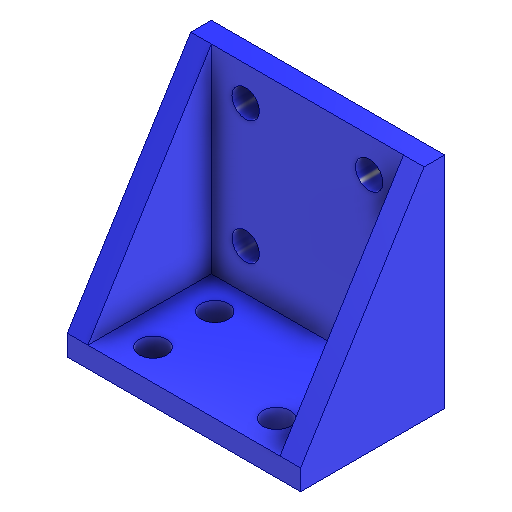
# Autodesk Inventor part: Escuadra
Saved by Autodesk Inventor 2025.3 (Build 293356000, 356)
## iProperties
Created: 2025-10-28
Part Number: Escuadra
Material: ABS Plastic
Document SubType Name: Modeling
Designer: Gabriel Bojaca
Density: 1.06 g/cm^3
Appearance: Blue - Wall Paint - Glossy
Author: Gabriel Bojaca
Title: Escuadra.ipt
Autodesk Inventor part; units mm, degrees
ref_plane "YZ Plane" through (0, 0, 0) normal (1, 0, 0) x (0, 1, 0)
ref_plane "XZ Plane" through (0, 0, 0) normal (0, 1, 0) x (-1, 0, 0)
ref_plane "XY Plane" through (0, 0, 0) normal (0, 0, 1) x (1, 0, 0)
sketch "Sketch1" plane through (0, 0, 0) normal (0, 0, 1) x (1, 0, 0)
  line L0 (-9, -9) -> (9, -9) construction
  line L1 (9, -9) -> (9, 9) construction
  line L2 (9, 9) -> (-9, 9) construction
  line L3 (-9, 9) -> (-9, -9) construction
  line L4 (-9, -9) -> (9, 9) construction
  line L5 (9, -9) -> (-9, 9) construction
  circle A0 centre (-9, 9) radius 2
  circle A1 centre (9, 9) radius 2
  circle A2 centre (9, -9) radius 2
  circle A3 centre (-9, -9) radius 2
  line L6 (-13.4025, 9) -> (21.0308, 9) construction
  line L7 (-13.4025, -18) -> (21.0308, -18)
  line L8 (14, -14) -> (-14, -14)
  line L9 (-14, -14) -> (-14, 14)
  line L10 (-14, 14) -> (14, 14)
  line L11 (14, 14) -> (14, -14)
  line L12 (-14, 14) -> (14, 14)
  line L13 (14, 14) -> (14, -18)
  line L14 (14, -18) -> (-14, -18)
  line L15 (-14, -18) -> (-14, 14)
  point P0 (0, 0)
  dimension "d0" = 18
  dimension "d1" = 18
  dimension "d2" = 4
  dimension "d3" = 4
  dimension "d4" = 27
  dimension "d5" = 5
  dimension "d6" = 9
  dimension "d7" = 14
  constraints: 32 end point, 7 parallel, 4 centre point, 3 horizontal, 3 perpendicular, 2 coincident, 2 midpoint, 2 symmetric about line, 1 point on line, 5 other
  measures "d0" distance of L2.end L1.end
  measures "d1" distance of L1.end L0.end
  measures "d2" diameter of A0
  measures "d3" diameter of A1
  measures "d4" distance between parallel lines of L6 L7
  measures "d5" distance between parallel lines of L0 L8
  measures "d6" distance from line of point (0, 0) L6
  measures "d7" distance from line of L9 point (0, 0)
extrude "Extrusion1" add sketch "Sketch1" along normal blind 3
sketch "Sketch2" plane through (-14, -18, 0) normal (0, -1, 0) x (1, 0, 0)
  line L0 (0, 3) -> (28, 3)
  line L1 (28, 3) -> (28, 21)
  line L2 (28, 21) -> (0, 21)
  line L3 (0, 21) -> (0, 3)
  line L4 (0, 21) -> (28, 3) construction
  line L5 (5, 7.5) -> (23, 7.5) construction
  line L6 (23, 7.5) -> (23, 16.5) construction
  line L7 (23, 16.5) -> (5, 16.5) construction
  line L8 (5, 16.5) -> (5, 7.5) construction
  line L9 (5, 7.5) -> (23, 16.5) construction
  line L10 (23, 7.5) -> (5, 16.5) construction
  circle A0 centre (5, 16.5) radius 2
  circle A1 centre (23, 16.5) radius 2
  line L11 (5, 12) -> (23, 12) construction
  line L12 (14, 16.5) -> (14, 7.5) construction
  circle A2 centre (5, 7.5) radius 2
  circle A3 centre (23, 7.5) radius 2
  line L13 (0, 0) -> (28, 0) projected
  line L14 (28, 0) -> (28, 3) projected
  line L15 (0, 3) -> (28, 3) projected
  line L16 (0, 0) -> (0, 3) projected
  line L17 (0, 0) -> (28, 0)
  line L18 (28, 0) -> (28, 3)
  line L19 (28, 3) -> (0, 3)
  line L20 (0, 3) -> (0, 0)
  point P0 (14, 0)
  point P1 (14, 12)
  dimension "d11" = 18
  dimension "d12" = 18
  dimension "d13" = 9
  dimension "d14" = 4
  dimension "d15" = 4
  constraints: 34 end point, 7 midpoint, 6 parallel, 4 centre point, 3 horizontal, 3 perpendicular, 2 coincident, 2 symmetric about line, 5 other
  measures "d11" distance of L1.end L0.end
  measures "d12" distance of L7.end L6.end
  measures "d13" distance of L6.end L5.end
  measures "d14" diameter of A0
  measures "d15" diameter of A1
extrude "Extrusion2" add sketch "Sketch2" against normal blind 3
sketch "Sketch4" plane through (-14, 14, 0) normal (-1, 0, 0) x (0, 0, 1)
  line L0 (3, -29) -> (3, 0) projected
  line L1 (21, -32) -> (21, -29) projected
  line L2 (0, 0) -> (0, -32) projected
  line L3 (3, -29) -> (21, -29) projected
  line L4 (21, -32) -> (21, -29) projected
  line L5 (3, 0) -> (3, -29) projected
  line L6 (0, 0) -> (3, 0) projected
  line L7 (0, -32) -> (21, -32) projected
  line L8 (3, 0) -> (21, -29)
  point P0 (0, -14)
  point P1 (3, -32)
  point P2 (3, 0)
  point P3 (21, -32)
  point P4 (3, 0)
  constraints: 2 end point
extrude "Extrusion3" add sketch "Sketch4" along normal blind 3
mirror "Mirror1" about plane through (0, 0, 0) normal (1, 0, 0) of "Extrusion3"
sketch "Sketch5" plane through (-14, -18, 0) normal (0, -1, 0) x (1, 0, 0)
  circle A0 centre (5, 7.5) radius 2 projected
  circle A1 centre (5, 7.5) radius 3
  point P0 (14, 0)
  dimension "d22" = 6
  constraints: 1 centre point, 1 coincident
  measures "d22" diameter of A1
sketch "Sketch6" plane through (0, 0, 3) normal (0, 0, 1) x (1, 0, 0)
  circle A0 centre (-9, -9) radius 2 projected
  circle A1 centre (-9, -9) radius 3
  point P0 (0, 0)
  dimension "d23" = 6
  constraints: 1 centre point, 1 coincident
  measures "d23" diameter of A1
body "Solid1"
